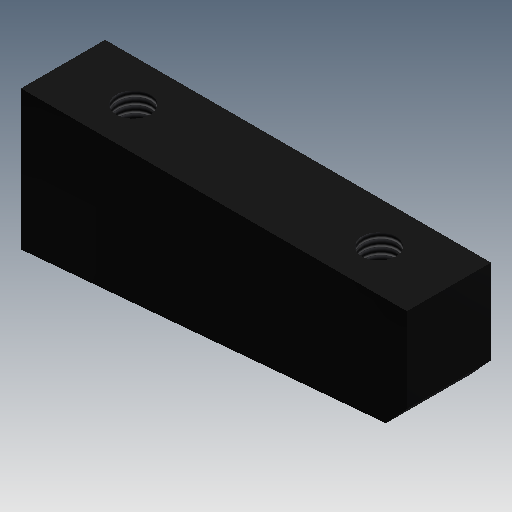
# Autodesk Inventor part: 210-105c
Saved by Autodesk Inventor 2020.1 (Build 241239000, 239)
## iProperties
Company: AUTODESK, INC.
Shininess: 64.0
Length Units: 11269
Angle Units: 11279
Time Units: 11290
Mass Units: 11283
Length Display Precision: 3
Angle Display Precision: 2
Compacted: True
Part Number: 210-105c
Document SubType Name: Modeling
Created: 2004-04-06
Designer: SCHNEIDER K.
Material: STEEL - HIGH GRADE ALLOY, BLACK OXIDE FINISH
Project: ADSK-000-000000
Description: GRIP PAD, TYPE-1
Density: 7.86 g/cm^3
Appearance: Glossy - Black
Density: 0.0
Volumn: 0.0
Area: 0.0
PropertySet Name: Model Information
Control State: 0
Master: False
Checked Out: False
Title: BLOCK
Author: SCHNEIDER K.
Revision Number: -
Autodesk Inventor part; units mm, degrees
ref_plane "YZ Plane" through (0, 0, 0) normal (1, 0, 0) x (0, 1, 0)
sketch "スケッチ2" plane through (0, 0, 0) normal (0, 0, 1) x (1, 0, 0)
  line L0 (-43.0479, 13.0453) -> (-43.0479, -8.9547)
  line L1 (-43.0479, -8.9547) -> (11.9521, -8.9547)
  line L2 (11.9521, -8.9547) -> (11.9521, 13.0453)
  line L3 (11.9521, 13.0453) -> (-43.0479, 13.0453)
  point P0 (0, 0)
  dimension "d3" = 55
  dimension "d16" = 22
  constraints: 9 end point
  measures "d3" distance between parallel lines of L2 L0
  measures "d16" distance of L1.end L2.end
extrude "押し出し2" add sketch "スケッチ2" along normal blind 12
sketch "スケッチ4" plane through (-43.0479, 13.0453, 0) normal (0, 1, 0) x (1, 0, 0)
  line L0 (55, 0) -> (55, -12) projected
  line L1 (0, 0) -> (0, -12) projected
  line L2 (0, -6) -> (55, -6)
  line L3 (0, -12) -> (55, -12) projected
  line L4 (0, 0) -> (55, 0) projected
  point P0 (10, -6)
  point P1 (45, -6)
  dimension "d17" = 10
  dimension "d18" = 35
  constraints: 2 end point, 2 midpoint, 2 point on line
  measures "d17" distance from line of point (10, -6) L1
  measures "d18" distance of point (45, -6) point (10, -6)
hole "穴2" at (-33.0479, 13.0453, 6) at (1.9521, 13.0453, 6) direction (0, -1, 0) diameter 4.917 depth 12 tip angle 118 thread size "M6x1" class "6H" standard "ISO Metric profile"
ref_plane "IN" through (-43.0479, -7.6232, 0) normal (-0.0872, 0.9962, 0) x (0, 0, 1)
ref_plane "OUT" through (-43.1176, -6.8262, 0) normal (-0.0872, 0.9962, 0) x (0, 0, 1)
sketch "スケッチ6" plane through (-43.1176, -6.8262, 0) normal (-0.0872, 0.9962, 0) x (0, 0, 1)
  line L0 (15.0202, 58.9603) -> (-3.3874, 58.9603)
  line L1 (-3.3874, 58.9603) -> (-3.3874, -4.1514)
  line L2 (-3.3874, -4.1514) -> (15.0202, -4.1514)
  line L3 (15.0202, -4.1514) -> (15.0202, 58.9603)
  constraints: 8 end point, 2 parallel, 1 horizontal, 1 perpendicular
extrude "押し出し4" cut sketch "スケッチ6" against normal through all
chamfer "面取り1" distance 3 angle 45 1 edges at (11.9521, -2.0083, 6)
body "Solid1"
